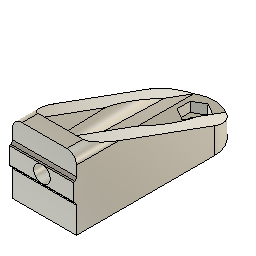
PU support 2 v3 (Autodesk Fusion 360 design; units mm, degrees)
Autodesk Fusion 360 part; units mm, degrees
note: some values were not read from the file. Chosen so that the rebuilt part matches the saved one: which face or edge a step refers to; which sketch regions a step uses.
sketch "Sketch1" plane through (0, 0, 0) normal (0, 1, 0) x (1, 0, 0)
  line L0 (0, 0) -> (20, 0)
  line L1 (20, 0) -> (20, -22)
  line L2 (20, -22) -> (0, -22)
  line L3 (0, -22) -> (0, 0)
  circle A0 centre (10, -12) radius 2.6
  circle A1 centre (10, -12) radius 5.5
  point P0 (10, -12)
  dimension "d1" = 20
  dimension "d2" = 22
  dimension "d3" = 10
  dimension "d4" = 5.2
  dimension "d5" = 11
  constraint horizontal L0
  constraint vertical L1
  constraint horizontal L2
  constraint vertical L3
  constraint coincident L0.start L3.end
  constraint coincident P0 A0.centre
  constraint concentric A0 A1
  measures "d1" distance of L0.start L0.end
  measures "d2" distance of L0.start L2.end
  measures "d3" distance of L2 P0
  measures "d4" diameter of A0
  measures "d5" diameter of A1
  measures "d59" diameter of P0
sketch "Sketch2" plane through (0, 0, 0) normal (1, 0, 0) x (0, 1, 0)
sketch "Sketch3" plane through (0, 0, 0) normal (0, 0, 1) x (1, 0, 0)
  line L0 (0, 0) -> (0, 43)
  line L1 (20, 0) -> (20, 43)
  line L2 (0, 0) -> (20, 0) construction
  line L3 (10, 0) -> (10, 31) construction
  line L4 (20, 0) -> (0, 0) construction
  arc A0 (20, 43) -> (0, 43) centre (10, 43) ccw
  line L5 (0, 5) -> (20, 5)
  line L6 (5, 5) -> (5, 51.6603)
  line L7 (15, 5) -> (15, 51.6603)
  line L8 (13.5, 49.0207) -> (10, 51.0415)
  line L9 (10, 51.0415) -> (6.5, 49.0207)
  line L10 (6.5, 49.0207) -> (6.5, 44.9793)
  line L11 (6.5, 44.9793) -> (10, 42.9585)
  line L12 (10, 42.9585) -> (13.5, 44.9793)
  line L13 (13.5, 44.9793) -> (13.5, 49.0207)
  circle A1 centre (10, 47) radius 2.1
  line L14 (20, 5) -> (20, 43)
  point P0 (0, 31)
  point P1 (20, 0)
  point P2 (10, 47)
  point P3 (10, 43)
  point P4 (10, 47)
  dimension "d8" = 47
  dimension "d12" = 5
  dimension "d13" = 5
  dimension "d55" = 3.5
  dimension "d59" = 4.2
  dimension "d63" = 4
  dimension "d65" = 4.6603
  constraint coincident L0.start L2.start
  constraint coincident P1 L1.start
  constraint midpoint L2 L3.start
  constraint coincident L3 P4
  constraint coincident L3 P3
  constraint coincident P3 A0.centre
  constraint tangent L0 A0
  constraint perpendicular L3 L5
  constraint parallel L0 L6
  constraint coincident A0 L6.end
  constraint symmetric L3 L6.start L7.start
  constraint symmetric L3 L6.end L7.end
  constraint coincident L1 L5.end
  constraint coincident L0 L5.start
  constraint coincident L5 L6.start
  constraint coincident P4 P2
  constraint tangent A0 L14
  measures "d8" distance of P4 L4
  measures "d12" distance of L4 L5
  measures "d13" distance of L0 L6
  measures "d55" distance of P4 L13
  measures "d59" diameter of A1
  measures "d63" distance of P4 P3
  measures "d65" vertical distance of P4 L6.end
extrude "Extrude1" add sketch "Sketch1" along normal blind 5 contours L0 L1 L2 L3
extrude "Extrude2" add sketch "Sketch3" along normal blind 5 contours A0 L5 L6 L7 | L8 L9 L10 L11 L12 L13 | A1
extrude "Extrude3" add sketch "Sketch1" along normal blind 3 contours A1
extrude "Extrude4" add sketch "Sketch3" along normal blind 3 contours A1
extrude "Extrude5" add sketch "Sketch3" along normal blind 22 contours L0 A0 L5 L6 | L1 A0 L5 L7 L14
sketch "Sketch4" plane through (5, 0, 0) normal (1, 0, 0) x (0, 1, 0)
  line L0 (5, 5) -> (51.6603, 5)
  line L1 (51.6603, 5) -> (51.6603, 22)
  line L2 (51.6603, 22) -> (5, 22)
  line L3 (5, 22) -> (5, 14.2913)
  line L4 (5, 14.2913) -> (5, 9.7087)
  line L5 (5, 9.7087) -> (5, 5)
  line L6 (5, 22) -> (51.6603, 5)
  line L7 (5, 5) -> (51.6603, 5)
  line L8 (5, 5) -> (5, 22)
  constraint coincident L2.end L3.start
  constraint coincident L0.end L1.start
  constraint coincident L0.start L5.end
extrude "Extrude6" cut sketch "Sketch4" along normal blind 31.651 and the other way blind 15.559 contours L1 L2 L6
extrude "Extrude7" cut 1 faces at (14.5032, 3, 12.4024) along direction (0, 1, 0) through all draft 1
sketch "Sketch5" plane through (0, 0, 0) normal (0, -1, 0) x (1, 0, 0)
  circle A0 centre (10, 12) radius 2.6
  line L0 (20, 22) -> (0, 22)
  line L1 (0, 22) -> (0, 0)
  line L2 (0, 0) -> (20, 0)
  line L3 (20, 0) -> (20, 22)
  line L4 (20, 12) -> (0, 12) construction
  line L5 (0, 15) -> (20, 15)
  line L6 (0, 9) -> (20, 9)
  line L7 (0, 15) -> (0, 9)
  line L8 (20, 15) -> (20, 9)
  dimension "d30" = 3
  constraint perpendicular L1 L4
  constraint coincident L3 L4.start
  constraint coincident L1 L4.end
  constraint perpendicular L3 L5
  constraint coincident L1 L5.start
  constraint coincident L3 L5.end
  constraint symmetric L4 L5.start L6.start
  constraint symmetric L4 L5.end L6.end
  measures "d30" distance of L4 L5
extrude "Extrude8" add sketch "Sketch5" along normal blind 0.8 contours L1 L3 L5 L6 L7 L8
fillet "Fillet1" radius 0.4 1 edges at (10, -0.8, 15)
fillet "Fillet1" radius 0.4 1 edges at (10, -0.8, 9)
fillet "Fillet2" radius 1 1 edges at (10, 0, 15)
fillet "Fillet2" radius 1 1 edges at (10, 0, 9)
fillet "Fillet3" radius 3 2 edges at (0, 2.5, 22) (20, 2.5, 22)
extrude "Extrude9" cut sketch "Sketch3" along normal blind 3 draft 1 from surface at 2 contours L8 L9 L10 L11 L12 L13 | A1
extrude "Extrude10" cut sketch "Sketch3" along normal through all contours A1
fillet "Fillet5" radius 3 1 edges at (10, 5, 5)
